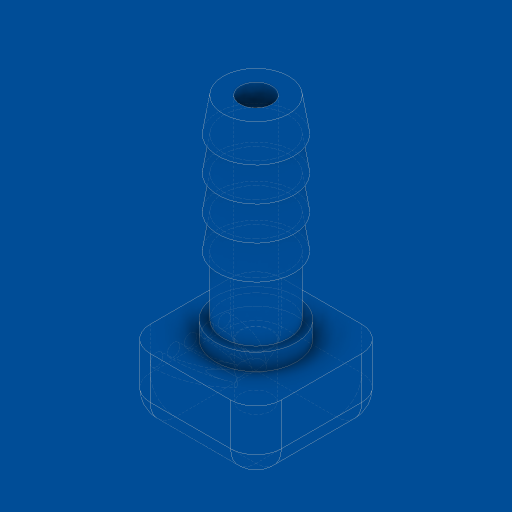
# Autodesk Inventor part: vacuum_vent
Saved by Autodesk Inventor 2023.2 (Build 272271000, 271)
## iProperties
Created: 2023-09-07
Part Number: vacuum_vent
Material: Generic
Document SubType Name: Modeling
Designer: agmlego
Mass: 2.72258 g
Surface Area: 20.5869 cm^2
Volume: 2.72258 cm^3
Density: 1 g/cm^3
Appearance: Default
Author: agmlego
Autodesk Inventor part; units mm, degrees
ref_plane "YZ Plane" through (0, 0, 0) normal (1, 0, 0) x (0, 1, 0)
ref_plane "XZ Plane" through (0, 0, 0) normal (0, 1, 0) x (-1, 0, 0)
sketch "Sketch2" plane through (0, 0, 0) normal (0, 0, 1) x (1, 0, 0)
  line L0 (0, 0) -> (0, 23)
  line L1 (1.875, 23) -> (1.875, 0)
  line L2 (1.875, 0) -> (3.875, 0)
  line L3 (3.875, 0) -> (3.875, 7)
  line L4 (3.875, 7) -> (4.5, 7)
  line L5 (4.5, 7) -> (3.875, 11)
  line L6 (3.875, 11) -> (4.5, 11)
  line L7 (4.5, 11) -> (3.875, 15)
  line L8 (3.875, 15) -> (4.5, 15)
  line L9 (4.5, 15) -> (3.875, 19)
  line L10 (3.875, 19) -> (4.5, 19)
  line L11 (4.5, 19) -> (3.875, 23)
  line L12 (3.875, 23) -> (1.875, 23)
  line L13 (3.875, 23) -> (3.875, 7) construction
  line L14 (4.5, 19) -> (4.5, 7) construction
  line L15 (-1.875, 23) -> (-1.875, 0) construction
  line L16 (-1.875, 0) -> (-3.875, 0) construction
  line L17 (-3.875, 0) -> (-3.875, 7) construction
  line L18 (-3.875, 7) -> (-4.5, 7) construction
  line L19 (-4.5, 7) -> (-3.875, 11) construction
  line L20 (-3.875, 11) -> (-4.5, 11) construction
  line L21 (-4.5, 11) -> (-3.875, 15) construction
  line L22 (-3.875, 15) -> (-4.5, 15) construction
  line L23 (-4.5, 15) -> (-3.875, 19) construction
  line L24 (-3.875, 19) -> (-4.5, 19) construction
  line L25 (-4.5, 19) -> (-3.875, 23) construction
  line L26 (-3.875, 23) -> (-1.875, 23) construction
  line L27 (-3.875, 23) -> (-3.875, 7) construction
  line L28 (-4.5, 19) -> (-4.5, 7) construction
  dimension "d0" = 23
  dimension "d1" = 7.75
  dimension "d2" = 9
  dimension "d3" = 2
  dimension "d4" = 4
  constraints: 58 end point, 14 point on line, 12 symmetric about line, 7 parallel, 3 perpendicular, 3 vertical, 1 midpoint
  measures "d0" distance between parallel lines of L2 L12
  measures "d1" distance between parallel lines of L17 L3
  measures "d2" distance between parallel lines of L14 L28
  measures "d3" distance of L1.end L2.end
  measures "d4" distance between parallel lines of L10 L12
revolve "Revolution1" add sketch "Sketch2" angle 360 about axis through (0, 0, 0) along (0, 1, 0)
sketch "Sketch5" plane through (0, 0, 0) normal (0, -1, 0) x (1, 0, 0)
  circle A0 centre (0, 0) radius 4.7625
  circle A1 centre (0, 0) radius 1.875 projected
  dimension "d6" = 9.525
  constraints: 1 centre point, 1 coincident
  measures "d6" diameter of A0
extrude "Extrusion1" add sketch "Sketch5" along normal blind 2
sketch "Sketch6" plane through (0, 0, 0) normal (0, 0, 1) x (1, 0, 0)
  line L0 (7.7625, -2) -> (-7.7625, -2)
  line L1 (-7.7625, -2) -> (-7.7625, -10)
  line L2 (-7.7625, -10) -> (7.7625, -10)
  line L3 (7.7625, -10) -> (7.7625, -2)
  line L4 (-4.7625, -2) -> (4.7625, -2) construction
  point P0 (0, 0)
  point P1 (0, -2)
  dimension "d9" = 8
  dimension "d10" = 3
  dimension "d11" = 15.525
  constraints: 8 end point, 2 midpoint, 2 parallel, 1 horizontal, 1 perpendicular
  measures "d9" distance of L2.end L0.start
  measures "d10" distance from line of L4.end L3
  measures "d11" distance of L1.end L2.end
extrude "Extrusion2" add sketch "Sketch6" along normal mid plane 15.525
sketch "Sketch7" plane through (0, -2, 0) normal (0, 1, 0) x (1, 0, 0)
  circle A0 centre (0, 0) radius 1.875 construction
  point P0 (0, 0)
  constraints: 1 coincident
hole "Hole1" at (0, -2, 0) direction (0, -1, 0) diameter 3.5719 depth 6.5
sketch "Sketch8" plane through (-7.7625, -10, 7.7625) normal (-1, 0, 0) x (0, 0, 1)
  line L0 (-15.525, 0) -> (0, 0) construction
  line L1 (0, 8) -> (0, 0) construction
  line L2 (0, 8) -> (-15.525, 8) construction
  line L3 (-15.525, 0) -> (-15.525, 8) construction
  line L4 (0, 8) -> (0, 0) construction
  line L5 (0, 4) -> (-15.525, 4) construction
  line L6 (-15.525, 0) -> (-15.525, 8) construction
  circle A0 centre (-11.7625, 4) radius 0.75
  circle A1 centre (-9.7625, 4) radius 0.75
  circle A2 centre (-7.7625, 4) radius 0.75
  circle A3 centre (-5.7625, 4) radius 0.75
  circle A4 centre (-3.7625, 4) radius 0.75
  point P0 (-7.7625, 10)
  point P1 (-7.7625, 4)
  dimension "d21" = 1.5
  dimension "d24" = 2
  constraints: 5 centre point, 3 midpoint, 2 end point, 1 coincident, 1 horizontal, 1 point on line, 8 other
  measures "d21" diameter of A0
  measures "d24" distance of A0.centre A1.centre
ref_plane "Work Plane1" through (-7.7625, -6, 7.7625) normal (0, -1, 0) x (1, 0, 0)
sketch "Sketch9" plane through (-7.7625, -6, 7.7625) normal (0, -1, 0) x (1, 0, 0)
  circle A0 centre (7.7625, -7.7625) radius 1.7859 construction
  circle A1 centre (7.7625, -7.7625) radius 1.7859 construction
  line L0 (7.7625, -7.7625) -> (0, -7.7625)
  arc A2 (7.7625, -7.7625) -> (0, -5.7625) centre (0, -21.8266) ccw
  arc A3 (0, -9.7625) -> (7.7625, -7.7625) centre (0, 6.3016) ccw
  arc A4 (0, -11.7625) -> (7.7625, -7.7625) centre (0, -2.2304) ccw
  arc A5 (7.7625, -7.7625) -> (0, -3.7625) centre (0, -13.2946) ccw
  line L1 (0, -15.525) -> (0, 0) construction
  constraints: 8 point on circle, 4 centre point, 4 line through centre, 2 end point, 1 horizontal
sweep "Sweep1" cut profiles "Sketch8" path "Sketch9" path curves L0 contours A2
sweep "Sweep2" cut profiles "Sketch8" path "Sketch9" path curves A3 contours A1
sweep "Sweep3" cut profiles "Sketch8" path "Sketch9" path curves A4 contours A0
sweep "Sweep4" cut profiles "Sketch8" path "Sketch9" path curves A2 contours A3
sweep "Sweep5" cut profiles "Sketch8" path "Sketch9" path curves A5 contours A4
fillet "Fillet1" radius 3 8 edges at (7.7625, -6, 7.7625) (7.7625, -6, -7.7625) (-7.7625, -6, -7.7625) (-7.7625, -6, 7.7625) (-7.7625, -10, 0) (0, -10, -7.7625) (7.7625, -10, 0) (0, -10, 7.7625)
equation "\"d12\" = d11"
body "Solid1"
